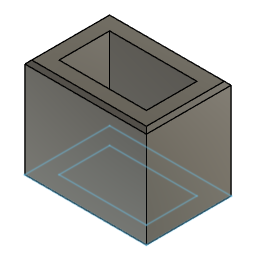
dispenser_axle_adapter_frankfork_arsenal (Autodesk Fusion 360 archive; units mm, degrees)
design "moottorinpää"
Autodesk Fusion 360 part; units mm, degrees
sketch "Sketch1" plane through (0, 0, 0) normal (0, 0, 1) x (1, 0, 0)
  line L0 (6.4875, 6.2322) -> (13.5875, 6.2322)
  line L1 (13.5875, 6.2322) -> (13.5875, 1.2822)
  line L2 (13.5875, 1.2822) -> (6.4875, 1.2822)
  line L3 (6.4875, 1.2822) -> (6.4875, 6.2322)
  line L4 (7.4875, 5.2322) -> (12.5875, 5.2322)
  line L5 (12.5875, 5.2322) -> (12.5875, 2.2822)
  line L6 (12.5875, 2.2822) -> (7.4875, 2.2822)
  line L7 (7.4875, 2.2822) -> (7.4875, 5.2322)
  dimension "d2" = 5.1
  dimension "d5" = 1
  dimension "d6" = 1
  dimension "d7" = 1
  dimension "d8" = 1
  dimension "d13" = 2.95
  constraint horizontal L0
  constraint vertical L1
  constraint horizontal L2
  constraint vertical L3
  constraint horizontal L4
  constraint vertical L5
  constraint horizontal L6
  constraint vertical L7
  measures "d2" distance of L4.start L4.end
  measures "d5" distance of L0 L4
  measures "d6" distance of L2 L6
  measures "d7" distance of L1 L5
  measures "d8" distance of L3 L7
  measures "d13" distance of L4 L6
extrude "Extrude1" add sketch "Sketch1" along normal blind 5.8
chamfer "Chamfer1" distance 0.2 angle 45 4 edges at (10.0375, 1.2822, 5.8) (13.5875, 3.7572, 5.8) (10.0375, 6.2322, 5.8) (6.4875, 3.7572, 5.8)
extrude "Extrude2" [suppressed]

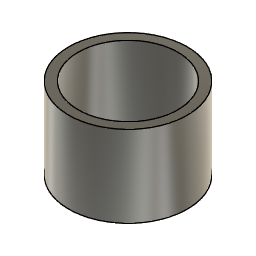
design "sirottimen pää"
Autodesk Fusion 360 part; units mm, degrees
sketch "Sketch1" plane through (0, 0, 0) normal (0, 0, 1) x (1, 0, 0)
  circle A0 centre (7, 3) radius 5.325
  circle A1 centre (7, 3) radius 6.325
  dimension "d1" = 10.65
  dimension "d3" = 1
  constraint concentric A0 A1
  measures "d1" diameter of A0
  measures "d3" distance of A0 A1
extrude "Extrude1" add sketch "Sketch1" along normal blind 8.69
